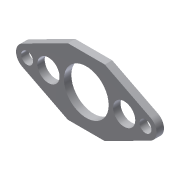
# Autodesk Inventor part: CIM Spacer
Saved by Autodesk Inventor 2013 (Build 170138000, 138)
## iProperties
Created: 2013-02-04
Part Number: CIM Spacer
Material: Aluminum 6061
Document SubType Name: Modeling
Designer: Niemitalo_Dan
Density: 1 g/cm^3
Author: Niemitalo_Dan
Autodesk Inventor part; units mm, degrees
ref_plane "YZ Plane" through (0, 0, 0) normal (1, 0, 0) x (0, 1, 0)
ref_plane "XZ Plane" through (0, 0, 0) normal (0, 1, 0) x (-1, 0, 0)
ref_plane "XY Plane" through (0, 0, 0) normal (0, 0, 1) x (1, 0, 0)
sketch "Sketch1" plane through (0, 0, 0) normal (0, 0, 1) x (1, 0, 0)
  circle A0 centre (0, 0) radius 9.6012
  circle A1 centre (-16.256, 0) radius 4.7625
  circle A2 centre (16.256, 0) radius 4.7625
  line L0 (7.9375, 14.224) -> (-7.9375, 14.224)
  line L1 (-7.9375, 14.224) -> (-27.5622, 4.2576)
  circle A3 centre (-25.4, 0) radius 2.5527
  arc A4 (-27.5622, 4.2576) -> (-27.5622, -4.2576) centre (-25.4, 0) ccw
  line L2 (-27.5622, -4.2576) -> (-7.9375, -14.224)
  line L3 (-7.9375, -14.224) -> (7.9375, -14.224)
  circle A5 centre (25.4, 0) radius 2.5527
  arc A6 (27.5622, -4.2576) -> (27.5622, 4.2576) centre (25.4, 0) ccw
  line L4 (7.9375, 14.224) -> (27.5622, 4.2576)
  line L5 (27.5622, -4.2576) -> (7.9375, -14.224)
  point P0 (0, 14.224)
  point P1 (0, -14.224)
  dimension "d0" = 19.2024
  dimension "d1" = 9.525
  dimension "d2" = 16.256
  dimension "d3" = 16.256
  dimension "d4" = 15.875
  dimension "d5" = 5.1054
  dimension "d6" = 25.4
  dimension "d7" = 4.7752
  dimension "d8" = 28.448
  dimension "d9" = 5.1054
  dimension "d10" = 25.4
  dimension "d11" = 4.7752
  dimension "d12" = 14.224
  constraints: 12 end point, 7 centre point, 4 horizontal alignment, 4 point on circle, 4 tangent, 3 coincident, 2 midpoint, 2 parallel, 2 vertical alignment, 1 equal radius, 1 horizontal
  measures "d0" diameter of A0
  measures "d1" diameter of A1
  measures "d2" distance of point (0, 0) A1.centre
  measures "d3" distance of A2.centre point (0, 0)
  measures "d4" distance of L0.start L0.end
  measures "d5" diameter of A3
  measures "d6" distance of A3.centre point (0, 0)
  measures "d7" radius of A4
  measures "d8" distance between parallel lines of L3 L0
  measures "d9" diameter of A5
  measures "d10" distance of A5.centre point (0, 0)
  measures "d11" radius of A6
  measures "d12" distance from line of L0 point (0, 0)
extrude "Extrusion1" add sketch "Sketch1" along normal blind 3.175
equation "\"d3\" = d2"
equation "\"d10\" = d6"
equation "\"d12\" = 0.5 * d8"
body "Solid1"
